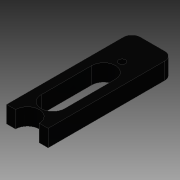
# Autodesk Inventor part: Fixture_Slide_Lock_Plate
Saved by Autodesk Inventor 2015 SP1 (Build 190203100, 203)
## iProperties
Created: 2014-12-16
Part Number: Fixture_Slide_Lock_Plate
Material: Generic
Document SubType Name: Modeling
Designer: amarschn
Density: 1 g/cm^3
Appearance: Anodized - Black
Author: amarschn
Autodesk Inventor part; units mm, degrees
ref_plane "YZ Plane" through (0, 0, 0) normal (1, 0, 0) x (0, 1, 0)
ref_plane "XZ Plane" through (0, 0, 0) normal (0, 1, 0) x (-1, 0, 0)
ref_plane "XY Plane" through (0, 0, 0) normal (0, 0, 1) x (1, 0, 0)
sketch "Sketch1" plane through (0, 0, 0) normal (0, 1, 0) x (-1, 0, 0)
  line L0 (-9.2075, -46.99) -> (9.2075, -46.99)
  line L1 (15.5575, -40.64) -> (15.5575, 46.99)
  line L2 (-15.5575, 46.99) -> (-15.5575, -40.64)
  line L3 (-15.5575, -46.99) -> (15.5575, 46.99) construction
  line L4 (15.5575, -46.99) -> (-15.5575, 46.99) construction
  circle A0 centre (0, -24.13) radius 2.54
  line L5 (8.89, -10.2337) -> (8.89, 27.8663)
  line L6 (-8.89, 27.8663) -> (-8.89, -10.2337)
  line L7 (-8.89, -10.2337) -> (8.89, 27.8663) construction
  line L8 (8.89, -10.2337) -> (-8.89, 27.8663) construction
  arc A1 (8.89, 27.8663) -> (-8.89, 27.8663) centre (0, 27.8663) ccw
  arc A2 (-8.89, -10.2337) -> (8.89, -10.2337) centre (0, -10.2337) ccw
  arc A3 (-8.89, 46.99) -> (8.89, 46.99) centre (0, 46.99) ccw
  line L9 (15.5575, 46.99) -> (8.89, 46.99)
  line L10 (-8.89, 46.99) -> (-15.5575, 46.99)
  arc A4 (9.2075, -46.99) -> (15.5575, -40.64) centre (9.2075, -40.64) ccw
  arc A5 (-15.5575, -40.64) -> (-9.2075, -46.99) centre (-9.2075, -40.64) ccw
  point P0 (0, 0)
  point P1 (0, 8.8163)
  dimension "d0" = 93.98
  dimension "d1" = 31.115
  dimension "d2" = 22.86
  dimension "d3" = 5.08
  dimension "d4" = 38.1
  dimension "d5" = 17.78
  dimension "d6" = 17.78
  dimension "d7" = 6.35
  constraints: 22 end point, 10 point on circle, 8 tangent, 6 centre point, 4 midpoint, 4 parallel, 4 point on line, 1 equal radius, 1 horizontal, 1 perpendicular
  measures "d0" distance of L4.start L1.end
  measures "d1" distance of L3.start L4.start
  measures "d2" distance from line of L0 A0.centre
  measures "d3" diameter of A0
  measures "d4" distance of A2.centre A1.centre
  measures "d5" distance between parallel lines of L6 L5
  measures "d6" diameter of A3
  measures "d7" radius of A4
extrude "Extrusion1" add sketch "Sketch1" along normal blind 12.7
equation "\"d6\" = d5"
body "Solid1"
